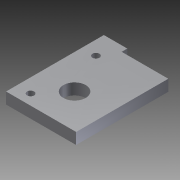
# Autodesk Inventor part: carro x lado motor pieza 2parte 2-3
Saved by Autodesk Inventor 2012 (Build 160160000, 160)
## iProperties
Created: 2014-12-17
Part Number: carro x lado motor pieza 2parte 2-3
Material: Default
Document SubType Name: Modeling
Designer: PRINCIPAL
Density: 1 g/cm^3
Author: PRINCIPAL
Autodesk Inventor part; units mm, degrees
ref_plane "YZ Plane" through (0, 0, 0) normal (1, 0, 0) x (0, 1, 0)
ref_plane "XZ Plane" through (0, 0, 0) normal (0, 1, 0) x (-1, 0, 0)
ref_plane "XY Plane" through (0, 0, 0) normal (0, 0, 1) x (1, 0, 0)
sketch "Boceto1" plane through (0, 0, 0) normal (0, 0, 1) x (1, 0, 0)
  arc A0 (-116.1173, -7.6512) -> (-117.6673, -9.2012) centre (-116.1173, -9.2012) ccw
  arc A1 (-117.6673, -9.2012) -> (-116.1173, -10.7512) centre (-116.1173, -9.2012) ccw
  arc A2 (-116.1173, -10.7512) -> (-114.5673, -9.2012) centre (-116.1173, -9.2012) ccw
  arc A3 (-114.5673, -9.2012) -> (-116.1173, -7.6512) centre (-116.1173, -9.2012) ccw
  arc A4 (-116.1173, -36.6512) -> (-117.6673, -38.2012) centre (-116.1173, -38.2012) ccw
  arc A5 (-117.6673, -38.2012) -> (-116.1173, -39.7512) centre (-116.1173, -38.2012) ccw
  arc A6 (-116.1173, -39.7512) -> (-114.5673, -38.2012) centre (-116.1173, -38.2012) ccw
  arc A7 (-114.5673, -38.2012) -> (-116.1173, -36.6512) centre (-116.1173, -38.2012) ccw
  arc A8 (-107.1173, -22.7512) -> (-112.0673, -27.7012) centre (-107.1173, -27.7012) ccw
  arc A9 (-112.0673, -27.7012) -> (-107.1173, -32.6512) centre (-107.1173, -27.7012) ccw
  arc A10 (-107.1173, -32.6512) -> (-102.1673, -27.7012) centre (-107.1173, -27.7012) ccw
  arc A11 (-102.1673, -27.7012) -> (-107.1173, -22.7512) centre (-107.1173, -27.7012) ccw
  line L0 (-91.2195, -2.0012) -> (-111.9173, -2.0012)
  line L1 (-111.9173, -2.0012) -> (-111.9173, 0.4988)
  line L2 (-111.9173, 0.4988) -> (-122.3173, 0.4988)
  line L3 (-122.3173, 0.4988) -> (-122.3173, -42.9012)
  line L4 (-122.3173, -42.9012) -> (-91.2195, -42.9012)
  line L5 (-91.2195, -42.9012) -> (-91.2195, -2.0012)
  point P0 (0, 0)
  constraints: 24 point on circle, 12 centre point, 12 end point
extrude "Extrusión1" add sketch "Boceto1" along normal blind 5
